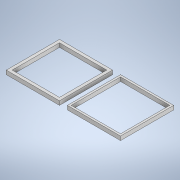
# Autodesk Inventor part: kwadrat
Saved by Autodesk Inventor 2020 (Build 240168000, 168)
## iProperties
Created: 2020-06-02
Part Number: kwadrat
Material: Generic
Document SubType Name: Modeling
Designer: atmat
Density: 1 g/cm^3
Appearance: Default
Author: atmat
Autodesk Inventor part; units mm, degrees
ref_plane "YZ Plane" through (0, 0, 0) normal (1, 0, 0) x (0, 1, 0)
ref_plane "XZ Plane" through (0, 0, 0) normal (0, 1, 0) x (-1, 0, 0)
ref_plane "XY Plane" through (0, 0, 0) normal (0, 0, 1) x (1, 0, 0)
sketch "Sketch1" plane through (0, 0, 0) normal (0, 1, 0) x (-1, 0, 0)
  line L0 (0, 0) -> (-13.5, 0)
  line L1 (-13.5, 0) -> (-13.5, -13.5)
  line L2 (-13.5, -13.5) -> (0, -13.5)
  line L3 (0, -13.5) -> (0, 0)
  line L4 (-12.75, -12.75) -> (-0.75, -12.75)
  line L5 (-0.75, -12.75) -> (-0.75, -0.75)
  line L6 (-0.75, -0.75) -> (-12.75, -0.75)
  line L7 (-12.75, -0.75) -> (-12.75, -12.75)
  line L8 (-15.5, -13.5) -> (-29, -13.5)
  line L9 (-29, -13.5) -> (-29, 0)
  line L10 (-29, 0) -> (-15.5, 0)
  line L11 (-15.5, 0) -> (-15.5, -13.5)
  line L12 (-16, -13) -> (-28.5, -13)
  line L13 (-28.5, -13) -> (-28.5, -0.5)
  line L14 (-28.5, -0.5) -> (-16, -0.5)
  line L15 (-16, -0.5) -> (-16, -13)
  dimension "d0" = 13.5
  dimension "d1" = 13.5
  dimension "d2" = 12
  dimension "d3" = 12
  dimension "d4" = 0.75
  dimension "d5" = 0.75
  dimension "d6" = 13.5
  dimension "d7" = 13.5
  dimension "d8" = 2
  dimension "d9" = 0.5
  dimension "d10" = 0.5
  dimension "d11" = 0.5
  dimension "d12" = 0.5
  dimension "d13" = 0
  constraints: 32 end point, 8 parallel, 4 horizontal, 4 perpendicular
  measures "d0" distance of L2.end L0.start
  measures "d1" distance of L0.start L0.end
  measures "d2" distance of L5.end L6.end
  measures "d3" distance of L6.end L4.start
  measures "d4" distance between parallel lines of L3 L5
  measures "d5" distance between parallel lines of L0 L6
  measures "d6" distance of L8.start L8.end
  measures "d7" distance of L10.end L8.start
  measures "d8" distance between parallel lines of L1 L11
  measures "d9" distance between parallel lines of L8 L12
  measures "d10" distance between parallel lines of L10 L14
  measures "d11" distance between parallel lines of L9 L13
  measures "d12" distance between parallel lines of L11 L15
  measures "d13" distance between parallel lines of L0 L10
extrude "Extrusion1" add sketch "Sketch1" along normal blind 1
body "Solid1"
